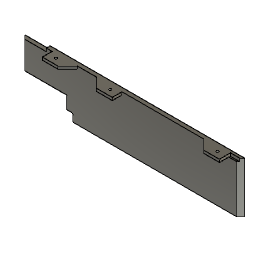
Side Wall v17 (Autodesk Fusion 360 design; units mm, degrees)
Autodesk Fusion 360 part; units mm, degrees
sketch "Sketch1" plane through (0, 0, 0) normal (0, 0, 1) x (1, 0, 0)
  line L0 (-92.95, 30) -> (190, 30)
  line L1 (190, 30) -> (190, 25)
  line L2 (190, 25) -> (-92.95, 25)
  line L3 (-92.95, 25) -> (-92.95, 30)
  circle A0 centre (-42.95, 20) radius 1.5
  circle A1 centre (27.05, 20) radius 1.5
  circle A2 centre (165, 20) radius 1.5
  line L4 (-52.95, 25) -> (-32.95, 25)
  line L5 (-32.95, 25) -> (-32.95, 12.5)
  line L6 (-32.95, 12.5) -> (-52.95, 12.5)
  line L7 (-52.95, 12.5) -> (-52.95, 25)
  line L8 (17.05, 25) -> (37.05, 25)
  line L9 (37.05, 25) -> (37.05, 12.5)
  line L10 (37.05, 12.5) -> (17.05, 12.5)
  line L11 (17.05, 12.5) -> (17.05, 25)
  line L12 (155, 25) -> (175, 25)
  line L13 (175, 25) -> (175, 12.5)
  line L14 (175, 12.5) -> (155, 12.5)
  line L15 (155, 12.5) -> (155, 25)
  line L16 (-92.95, 30) -> (-87.95, 25)
  line L17 (190, 30) -> (185, 25)
  line L18 (-32.95, 12.5) -> (-20.45, 25)
  line L19 (17.05, 12.5) -> (4.55, 25)
  line L20 (155, 12.5) -> (142.5, 25)
  dimension "d1" = 282.95
  dimension "d2" = 5
  dimension "d3" = 3
  dimension "d4" = 10
  dimension "d5" = 50
  dimension "d6" = 3
  dimension "d7" = 70
  dimension "d8" = 10
  dimension "d9" = 3
  dimension "d10" = 25
  dimension "d11" = 10
  dimension "d12" = 10
  dimension "d13" = 10
  dimension "d14" = 7.5
  dimension "d15" = 10
  dimension "d16" = 7.5
  dimension "d17" = 10
  dimension "d18" = 10
  dimension "d19" = 10
  dimension "d20" = 7.5
  dimension "d21" = 45
  dimension "d22" = 45
  dimension "d24" = 45
  dimension "d25" = 45
  dimension "d27" = 45
  dimension "d36" = 40
  constraint horizontal L0
  constraint vertical L1
  constraint horizontal L2
  constraint vertical L3
  constraint horizontal L4
  constraint vertical L5
  constraint horizontal L6
  constraint vertical L7
  constraint coincident L2 L4.start
  constraint horizontal L8
  constraint vertical L9
  constraint horizontal L10
  constraint vertical L11
  constraint coincident L2 L8.start
  constraint horizontal L12
  constraint vertical L13
  constraint horizontal L14
  constraint vertical L15
  constraint coincident L2 L12.start
  constraint coincident L2 L16.end
  constraint coincident L2 L17.end
  constraint coincident L2 L18.end
  constraint coincident L2 L19.end
  constraint coincident L2 L20.end
  measures "d1" distance of L1 L3
  measures "d2" distance of L0.start L2.end
  measures "d3" diameter of A0
  measures "d4" distance of L0 A0.centre
  measures "d5" distance of L3 A0.centre
  measures "d6" diameter of A1
  measures "d7" distance of A0.centre A1.centre
  measures "d8" distance of L0 A1.centre
  measures "d9" diameter of A2
  measures "d10" distance of L1 A2.centre
  measures "d11" distance of L0 A2.centre
  measures "d12" distance of A0.centre L7
  measures "d13" distance of A0.centre L5
  measures "d14" distance of A0.centre L6
  measures "d15" distance of A1.centre L11
  measures "d16" distance of A1.centre L10
  measures "d17" distance of A1.centre L9
  measures "d18" distance of A2.centre L15
  measures "d19" distance of A2.centre L13
  measures "d20" distance of A2.centre L14
  measures "d21" angle of L3 L16
  measures "d22" angle of L1 L17
  measures "d24" angle of L5 L18
  measures "d25" angle of L11 L19
  measures "d27" angle of L15 L20
  measures "d36" distance of L2.end L4.start
extrude "Extrude8" add sketch "Sketch1" against normal blind 3.5 contours L0 L2 L4 L8 L12 L16 L17 | L2 L4 L5 L6 L7 | L2 L12 L13 L14 L15 | L2 L5 L18 | L2 L15 L20 | L2 L11 L19 | L2 L8 L9 L10 L11
extrude "Extrude9" add sketch "Sketch1" against normal blind 65.5 contours L0 L2 L4 L8 L12 L16 L17
sketch "Sketch5" plane through (0, 0, 0) normal (0, 0, 1) x (1, 0, 0)
  line L0 (-92.95, 30) -> (-60.45, 30)
  line L1 (-60.45, 30) -> (-60.45, 25)
  line L2 (-60.45, 25) -> (-92.95, 25)
  line L3 (-92.95, 25) -> (-92.95, 30)
  line L4 (-92.95, 25) -> (-92.95, 30)
  line L5 (190, 30) -> (190, 25)
  line L6 (-92.95, 30) -> (190, 30)
  line L7 (190, 25) -> (175, 25)
  line L8 (175, 25) -> (175, 26.8)
  line L9 (175, 26.8) -> (190, 26.8)
  line L10 (190, 26.8) -> (190, 25)
  dimension "d54" = 250.45
  dimension "d55" = 32.5
  dimension "d56" = 5
  dimension "d64" = 1.8
  dimension "d65" = 15
  constraint horizontal L0
  constraint vertical L1
  constraint horizontal L2
  constraint vertical L3
  constraint horizontal L7
  constraint vertical L8
  constraint horizontal L9
  constraint vertical L10
  constraint coincident L5.end L7.start
  measures "d54" distance of L1 L5
  measures "d55" distance of L1 L3
  measures "d56" distance of L2 L6
  measures "d64" distance of L7 L9
  measures "d65" distance of L8 L10
extrude "Extrude10" cut sketch "Sketch5" against normal blind 4 contours L0 L1 L2 L3 L4 L6
sketch "Sketch7" plane through (0, 0, -65.5) normal (0, 0, -1) x (1, 0, 0)
  line L0 (-87.95, -25) -> (-92.95, -30)
  line L1 (-92.95, -30) -> (190, -30)
  line L2 (190, -30) -> (185, -25)
  line L3 (185, -25) -> (-87.95, -25)
  line L4 (-92.95, -30) -> (-34.15, -30)
  line L5 (-34.15, -30) -> (-34.15, -25)
  line L6 (-34.15, -25) -> (-92.95, -25)
  line L7 (-92.95, -25) -> (-92.95, -30)
  line L8 (-34.15, -30) -> (-26.15, -30)
  line L9 (-26.15, -30) -> (-26.15, -25)
  line L10 (-26.15, -25) -> (-34.15, -25)
  line L11 (-34.15, -25) -> (-34.15, -30)
  dimension "d60" = 5
  dimension "d61" = 58.8
  dimension "d68" = 8
  constraint horizontal L4
  constraint vertical L5
  constraint horizontal L6
  constraint vertical L7
  constraint coincident L3 L5.end
  constraint coincident L0.end L1.start
  constraint horizontal L8
  constraint vertical L9
  constraint horizontal L10
  constraint vertical L11
  constraint coincident L3 L9.end
  measures "d60" distance of L4 L6
  measures "d61" distance of L5 L7
  measures "d68" distance of L9 L11
extrude "Extrude11" cut sketch "Sketch7" against normal blind 26.25 contours L0 L1 L3 L4 L5 L6 L11
extrude "Extrude12" cut sketch "Sketch5" against normal blind 4 contours L5 L7 L8 L9 L10
extrude "Extrude13" cut sketch "Sketch7" against normal blind 10 contours L1 L3 L5 L8 L9 L10 L11
fillet "Fillet1" radius 2 1 edges at (-26.15, 27.5, -55.5)
